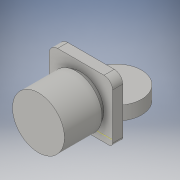
# Autodesk Inventor part: Light Circuit
Saved by Autodesk Inventor 2016 (Build 200138000, 138)
## iProperties
Created: 2017-12-20
Part Number: Light Circuit
Material: Generic
Document SubType Name: Modeling
Designer: Student
Density: 1 g/cm^3
Appearance: Default
Author: Student
Autodesk Inventor part; units mm, degrees
ref_plane "YZ Plane" through (0, 0, 0) normal (1, 0, 0) x (0, 1, 0)
ref_plane "XZ Plane" through (0, 0, 0) normal (0, 1, 0) x (-1, 0, 0)
ref_plane "XY Plane" through (0, 0, 0) normal (0, 0, 1) x (1, 0, 0)
sketch "Sketch1" plane through (0, 0, 0) normal (0, 0, 1) x (1, 0, 0)
  line L0 (-8.636, 11.7475) -> (8.636, 11.7475)
  line L1 (11.811, 8.5725) -> (11.811, -8.5725)
  line L2 (10.541, -9.8425) -> (-10.541, -9.8425)
  line L3 (-11.811, -8.5725) -> (-11.811, 8.5725)
  arc A0 (-8.636, 11.7475) -> (-11.811, 8.5725) centre (-8.636, 8.5725) ccw
  arc A1 (11.811, 8.5725) -> (8.636, 11.7475) centre (8.636, 8.5725) ccw
  arc A2 (-11.811, -8.5725) -> (-10.541, -9.8425) centre (-10.541, -8.5725) ccw
  arc A3 (10.541, -9.8425) -> (11.811, -8.5725) centre (10.541, -8.5725) ccw
  arc A4 (-11.811, -8.5725) -> (-10.541, -9.8425) centre (-10.541, -8.5725) ccw
  point P0 (0, 0)
  point P1 (0, 11.7475)
  point P2 (11.811, 0)
  dimension "d0" = 23.622
  dimension "d1" = 21.59
  dimension "d2" = 3.175
  dimension "d3" = 1.27
  dimension "d4" = 1.27
  constraints: 10 point on circle, 10 tangent, 8 end point, 5 centre point, 2 equal radius, 2 midpoint, 2 parallel, 2 point on line, 1 horizontal, 1 horizontal alignment, 1 perpendicular, 1 vertical alignment
  measures "d0" distance between parallel lines of L1 L3
  measures "d1" distance between parallel lines of L2 L0
  measures "d2" radius of A0
  measures "d3" radius of A2
  measures "d4" radius of A3
extrude "Extrusion1" add sketch "Sketch1" along normal blind 3.81
ref_plane "Work Plane1" through (-10.541, -7.3025, 0) normal (0, -1, 0) x (1, 0, 0)
sketch "Sketch2" plane through (-10.541, -7.3025, 0) normal (0, -1, 0) x (1, 0, 0)
  circle A0 centre (10.541, -9.398) radius 9.398
  line L0 (0, 0) -> (21.082, 0) projected
  point P0 (10.541, 0)
  point P1 (10.541, 0)
  dimension "d8" = 18.796
  constraints: 1 centre point, 1 midpoint, 1 tangent, 1 vertical alignment
  measures "d8" diameter of A0
extrude "Extrusion2" add sketch "Sketch2" against normal blind 5.08
sketch "Sketch3" plane through (0, 0, 3.81) normal (0, 0, 1) x (1, 0, 0)
  circle A0 centre (0, 0) radius 8.5489
  constraints: 1 centre point, 1 coincident
extrude "Extrusion3" add sketch "Sketch3" along normal blind 1.778
sketch "Sketch4" plane through (0, 0, 5.588) normal (0, 0, 1) x (1, 0, 0)
  circle A0 centre (0, 0) radius 9.6564
  constraints: 1 centre point, 1 coincident
extrude "Extrusion4" add sketch "Sketch4" along normal blind 13.97
body "Solid1"
